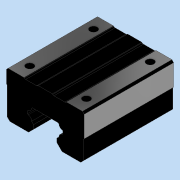
# Autodesk Inventor part: HGR20A
Saved by Autodesk Inventor 2021 (Build 250183000, 183)
## iProperties
Created: 2021-09-26
Part Number: HGR20A
Material: Generic
Document SubType Name: Modeling
Designer: 41601100
Density: 1 g/cm^3
Appearance: Default
Author: 41601100
Autodesk Inventor part; units mm, degrees
ref_plane "YZ Plane" through (0, 0, 0) normal (1, 0, 0) x (0, 1, 0)
ref_plane "XZ Plane" through (0, 0, 0) normal (0, 1, 0) x (-1, 0, 0)
ref_plane "XY Plane" through (0, 0, 0) normal (0, 0, 1) x (1, 0, 0)
sketch "Sketch1" plane through (0, 0, 0) normal (0, 0, 1) x (1, 0, 0)
  line L0 (-22, 15) -> (-22, 8)
  line L1 (-21, 16) -> (-22, 15)
  line L2 (-12, 16) -> (-21, 16)
  line L3 (-11.8, 15.8) -> (-12, 16)
  arc A0 (-11.8, 15.8) -> (-11.0859, 15.5) centre (-11.0859, 16.5) ccw
  line L4 (-4.9141, 15.5) -> (-11.0859, 15.5)
  arc A1 (-4.9141, 15.5) -> (-4.2, 15.8) centre (-4.9141, 16.5) ccw
  line L5 (-4, 16) -> (-4.2, 15.8)
  line L6 (4, 16) -> (-4, 16)
  line L7 (4.2, 15.8) -> (4, 16)
  arc A2 (4.2, 15.8) -> (4.9141, 15.5) centre (4.9141, 16.5) ccw
  line L8 (11.0859, 15.5) -> (4.9141, 15.5)
  arc A3 (11.0859, 15.5) -> (11.8, 15.8) centre (11.0859, 16.5) ccw
  line L9 (12, 16) -> (11.8, 15.8)
  line L10 (21, 16) -> (12, 16)
  line L11 (22, 15) -> (21, 16)
  line L12 (22, 3) -> (22, 15)
  line L13 (21.5, 2.5) -> (22, 3)
  line L14 (21.5, -8) -> (21.5, 2.5)
  line L15 (20, -9.5) -> (21.5, -8)
  line L16 (9.45, -9.5) -> (20, -9.5)
  line L17 (6.6, -6.65) -> (9.45, -9.5)
  line L18 (6.6, -4.35) -> (6.6, -6.65)
  line L19 (7.7, -3.25) -> (6.6, -4.35)
  arc A4 (9.6, -1.075) -> (7.7, -3.25) centre (9.8292, -3.1926) ccw
  line L20 (10, -0.675) -> (9.6, -1.075)
  line L21 (10, 0.675) -> (10, -0.675)
  line L22 (9.6, 1.075) -> (10, 0.675)
  arc A5 (7.7, 3.1) -> (9.6, 1.075) centre (9.828, 3.1928) ccw
  line L23 (7.3, 3.5) -> (7.7, 3.1)
  line L24 (-7.3, 3.5) -> (7.3, 3.5)
  line L25 (-7.7, 3.1) -> (-7.3, 3.5)
  arc A6 (-9.6, 1.075) -> (-7.7, 3.1) centre (-9.828, 3.1928) ccw
  line L26 (-10, 0.675) -> (-9.6, 1.075)
  line L27 (-10, -0.675) -> (-10, 0.675)
  line L28 (-9.6, -1.075) -> (-10, -0.675)
  arc A7 (-7.7, -3.25) -> (-9.6, -1.075) centre (-9.8292, -3.1926) ccw
  line L29 (-6.6, -4.35) -> (-7.7, -3.25)
  line L30 (-6.6, -6.65) -> (-6.6, -4.35)
  line L31 (-9.45, -9.5) -> (-6.6, -6.65)
  line L32 (-20, -9.5) -> (-9.45, -9.5)
  line L33 (-21.5, -8) -> (-20, -9.5)
  line L34 (-21.5, 7.5) -> (-21.5, -8)
  line L35 (-22, 8) -> (-21.5, 7.5)
  point P0 (0, 0)
  point P1 (0, 0)
  constraints: 72 end point, 16 point on circle, 8 centre point
extrude "Extrusion1" add sketch "Sketch1" against normal blind 50.5
sketch "Sketch3" plane through (-21, 16, 0) normal (0, 1, 0) x (1, 0, 0)
  line L0 (9, 50.5) -> (0, 50.5)
  line L1 (0, 0) -> (0, 50.5)
  line L2 (9, 0) -> (0, 0)
  line L3 (9, 0) -> (9, 50.5)
  circle A0 centre (5, 7.25) radius 2.1
  circle A1 centre (5, 43.25) radius 2.1
  line L4 (42, 50.5) -> (33, 50.5)
  line L5 (33, 0) -> (33, 50.5)
  line L6 (42, 0) -> (33, 0)
  line L7 (42, 0) -> (42, 50.5)
  circle A2 centre (37, 7.25) radius 2.1
  circle A3 centre (37, 43.25) radius 2.1
  line L8 (9, 0) -> (0, 0) projected
  line L9 (9, 0) -> (9, 50.5) projected
  line L10 (0, 50.5) -> (9, 50.5) projected
  line L11 (0, 0) -> (0, 50.5) projected
  line L12 (42, 0) -> (33, 0) projected
  line L13 (42, 0) -> (42, 50.5) projected
  line L14 (33, 50.5) -> (42, 50.5) projected
  line L15 (33, 0) -> (33, 50.5) projected
  point P0 (21, 0)
  point P1 (21, 25.25)
  constraints: 16 end point, 4 centre point
extrude "Extrusion2" cut sketch "Sketch3" against normal blind 6 contours A0 | A1 | A2 | A3
body "Solid1"
